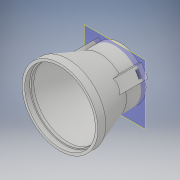
# Autodesk Inventor part: endkappen
Saved by Autodesk Inventor 2017 (Build 210142000, 142)
## iProperties
Part Number: endkappen
Material: Generisch
Document SubType Name: Modeling
Designer: Fabio
Density: 1 g/cm^3
Appearance: Vorgabe
Author: Fabio
Autodesk Inventor part; units mm, degrees
ref_plane "YZ Plane" through (0, 0, 0) normal (1, 0, 0) x (0, 1, 0)
ref_plane "XZ Plane" through (0, 0, 0) normal (0, 1, 0) x (-1, 0, 0)
ref_plane "XY Plane" through (0, 0, 0) normal (0, 0, 1) x (1, 0, 0)
sketch "Skizze2" plane through (0, 0, 0) normal (1, 0, 0) x (0, 1, 0)
  line L0 (47.4748, 12) -> (6.2626, 27)
  line L1 (0, 0) -> (48.6481, 0)
  line L2 (6.2626, 30) -> (0, 30)
  line L3 (6.2626, 27) -> (4, 27)
  line L4 (4, 27) -> (4, 28)
  line L5 (4, 28) -> (0, 28)
  line L6 (0, 0) -> (0, 28) construction
  line L7 (0, 28) -> (0, 30)
  line L8 (47.4748, 12) -> (47.4748, 20.6434)
  line L9 (47.4748, 20.6434) -> (31.9696, 20.6434)
  line L10 (6.2626, 30) -> (31.9696, 20.6434)
  dimension "d21" = 24
  dimension "d22" = 20
  dimension "d55" = 4
  dimension "d56" = 2
  dimension "d57" = 60
  dimension "d58" = 2.2626
  dimension "d59" = 1
  dimension "d60" = 6.2626
  dimension "d115" = 15.5052
  constraints: 22 end point, 4 horizontal, 2 perpendicular, 2 vertical, 1 collinear, 1 parallel
  measures "d21" diameter of L0.start L1
  measures "d22" angle of L1 L0
  measures "d55" distance of L4.end L5.end
  measures "d56" distance of L5.end L2.end
  measures "d57" diameter of L2 L1
  measures "d58" distance of L0.end L3.end
  measures "d59" distance of L3.end L4.end
  measures "d60" distance of L2.start L2.end
  measures "d115" distance of L8.end L9.end
revolve "Umdrehung1" add sketch "Skizze2" angle 360 about axis through (0, 0, 0) along (0, 1, 0)
sketch "Skizze15" plane through (0, 47.4748, 0) normal (0, 1, 0) x (1, 0, 0)
  circle A0 centre (0, 0) radius 20.6434 projected
  circle A1 centre (0, 0) radius 12 projected
  line L0 (-5, 18.6434) -> (-5, 22.6434)
  line L1 (-5, 22.6434) -> (5, 22.6434)
  line L2 (5, 22.6434) -> (5, 18.6434)
  line L3 (5, 18.6434) -> (-5, 18.6434)
  line L4 (-5, 18.6434) -> (5, 22.6434) construction
  line L5 (-5, 22.6434) -> (5, 18.6434) construction
  line L6 (-17.1098, -15.6518) -> (-22.1098, -6.9916)
  line L7 (-22.1098, -6.9916) -> (-18.6457, -4.9916)
  line L8 (-18.6457, -4.9916) -> (-13.6457, -13.6518)
  line L9 (-13.6457, -13.6518) -> (-17.1098, -15.6518)
  line L10 (22.1098, -6.9916) -> (17.1098, -15.6518)
  line L11 (17.1098, -15.6518) -> (13.6457, -13.6518)
  line L12 (13.6457, -13.6518) -> (18.6457, -4.9916)
  line L13 (18.6457, -4.9916) -> (22.1098, -6.9916)
  point P0 (0, 20.6434)
  dimension "d129" = 10
  dimension "d130" = 4
  dimension "d131" = 18.6434
  dimension "d134" = 360
  constraints: 28 end point, 2 midpoint, 2 parallel, 1 perpendicular, 1 vertical, 1 vertical alignment, 26 other
  measures "d129" distance of L0.end L1.end
  measures "d130" distance of L1.end L2.end
  measures "d131" distance from line of point (0, 0) L3
extrude "Extrusion12" add sketch "Skizze15" against normal blind 25 contours L2 L3 L0 A0 | A0 L0 L1 L2 | L13 L10 L11 A0 | A0 L11 L12 L13 | L7 L8 L9 A0 | A0 L9 L6 L7
delete faces "Fläche löschen5" heal yes whole lump no faces at (0, 24.7239, -18.6434) (-0.5603, 22.4748, -19.4397)
delete faces "Fläche löschen6" heal yes whole lump no faces at (16.5551, 22.4748, 10.2051) (16.1457, 24.7239, 9.3217)
delete faces "Fläche löschen7" heal yes whole lump no faces at (-17.1154, 22.4748, 9.2346) (-16.1457, 24.7239, 9.3217)
ref_plane "Arbeitsebene2" through (-5, 43.4748, -22.6434) normal (0, 1, 0) x (1, 0, 0)
sketch "Skizze16" plane through (-5, 43.4748, -22.6434) normal (0, 1, 0) x (1, 0, 0)
  line L0 (-17.1098, -29.635) -> (-12.1098, -38.2953) projected
  line L1 (0, 0) -> (10, 0) projected
  line L2 (2.15, 5.7) -> (7.85, 5.7)
  line L3 (7.85, 5.7) -> (7.85, -5.7)
  line L4 (7.85, -5.7) -> (2.15, -5.7)
  line L5 (2.15, -5.7) -> (2.15, 5.7)
  line L6 (2.15, 5.7) -> (7.85, -5.7) construction
  line L7 (7.85, 5.7) -> (2.15, -5.7) construction
  line L8 (-20.9711, -34.347) -> (-11.0984, -28.647)
  line L9 (-18.1211, -39.2833) -> (-20.9711, -34.347)
  line L10 (-8.2484, -33.5833) -> (-18.1211, -39.2833)
  line L11 (-11.0984, -28.647) -> (-8.2484, -33.5833)
  line L12 (28.1211, -39.2833) -> (18.2484, -33.5833)
  line L13 (30.9711, -34.347) -> (28.1211, -39.2833)
  line L14 (21.0984, -28.647) -> (30.9711, -34.347)
  line L15 (18.2484, -33.5833) -> (21.0984, -28.647)
  point P0 (5, -22.6434)
  point P1 (5, 0)
  dimension "d139" = 5.7
  dimension "d140" = 11.4
  dimension "d143" = 360
  constraints: 28 end point, 3 midpoint, 2 parallel, 1 horizontal, 1 perpendicular, 25 other
  measures "d139" distance of L3.end L4.end
  measures "d140" distance of L2.end L3.end
extrude "Extrusion13" cut sketch "Skizze16" against normal blind 2
sketch "Skizze17" plane through (-5, 47.4748, -22.6434) normal (0, 1, 0) x (1, 0, 0)
  line L0 (0, 0) -> (10, 0) projected
  line L1 (5, -22.6434) -> (5, -2.85) construction
  point P0 (-12.1416, -32.5402)
  point P1 (22.1416, -32.5402)
  dimension "d147" = 2.85
  dimension "d150" = 360
  constraints: 2 end point, 1 coincident, 1 vertical, 4 other
  measures "d147" distance from line of L0 L1.end
hole "Bohrung3" at (0, 47.4748, -19.7934) at (-17.1416, 47.4748, 9.8967) at (17.1416, 47.4748, 9.8967) direction (0, -1, 0) diameter 3.3 depth 15 tip angle 118
fillet "Rundung1" radius 2 1 edges at (0, 47.4748, -12)
